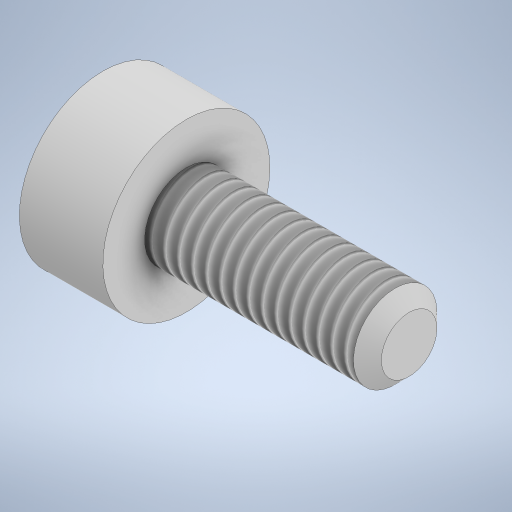
# Autodesk Inventor part: М3х8
Saved by Autodesk Inventor 2023 (Build 270158000, 158)
## iProperties
Created: 2022-05-02
Part Number: М3х8
Material: Типовые
Document SubType Name: Modeling
Designer: User
Density: 1 g/cm^3
Appearance: По умолчанию
Author: User
Autodesk Inventor part; units mm, degrees
ref_plane "YZ Plane" through (0, 0, 0) normal (1, 0, 0) x (0, 1, 0)
ref_plane "XZ Plane" through (0, 0, 0) normal (0, 1, 0) x (-1, 0, 0)
ref_plane "XY Plane" through (0, 0, 0) normal (0, 0, 1) x (1, 0, 0)
sketch "Эскиз1" plane through (0, 0, 0) normal (0, 0, 1) x (1, 0, 0)
  line L0 (0, 0) -> (0, 3)
  line L1 (0, 3) -> (3, 3)
  line L2 (3, 3) -> (3, 0)
  line L3 (3, 0) -> (11, 0)
  line L4 (11, 0) -> (11, 1.5)
  line L5 (11, 1.5) -> (3, 1.5)
  line L6 (0, 0) -> (3, 0)
  line L7 (3, 0) -> (0, 0)
  dimension "d0" = 3
  dimension "d1" = 3
  dimension "d2" = 8
  dimension "d3" = 1.5
  constraints: 16 end point, 4 perpendicular, 1 collinear, 1 midpoint, 1 parallel, 1 vertical
  measures "d0" distance of L0.start L0.end
  measures "d1" distance of L0.end L1.end
  measures "d2" distance of L2.end L3.end
  measures "d3" distance of L3.end L4.end
revolve "Вращение1" add sketch "Эскиз1" angle 360 about axis through (3, 0, 0) along (1, 0, 0)
thread "Резьба1" size "M3x0.5" class "6g" standard "ISO Metric profile" full length
chamfer "Фаска1" distance 0.5 angle 45 1 edges at (11, -1.5, 0)
